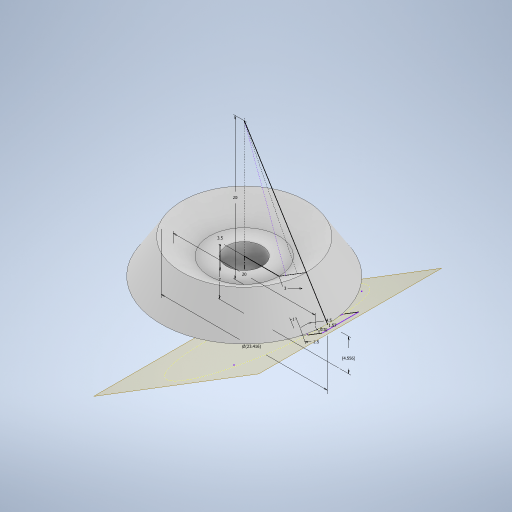
# Autodesk Inventor part: 베벨기어 002
Saved by Autodesk Inventor 2023 (Build 270158000, 158)
## iProperties
Created: 2022-06-18
Part Number: 베벨기어 002
Material: 일반
Document SubType Name: Modeling
Designer: fly01
Density: 1 g/cm^3
Appearance: 기본값
Author: fly01
Autodesk Inventor part; units mm, degrees
ref_plane "YZ Plane" through (0, 0, 0) normal (1, 0, 0) x (0, 1, 0)
ref_plane "XZ Plane" through (0, 0, 0) normal (0, 1, 0) x (-1, 0, 0)
ref_plane "XY Plane" through (0, 0, 0) normal (0, 0, 1) x (1, 0, 0)
sketch "스케치1" plane through (0, 0, 0) normal (0, 0, 1) x (1, 0, 0)
  line L0 (-10, 0) -> (10, 0) construction
  line L1 (0, 0) -> (0, 20) construction
  line L2 (0, 20) -> (10, 0) construction
  line L3 (0, 20) -> (11.7082, 1.0557)
  line L4 (0, 20) -> (5.8657, 4.0994) construction
  line L5 (7.8647, -1.3197) -> (11.7082, 1.0557)
  line L6 (7.8647, -1.3197) -> (7.0141, -1.8454)
  line L7 (7.0141, -1.8454) -> (3.9324, -1.8454)
  line L8 (3.9324, -1.8454) -> (3.9324, -3.5)
  line L9 (3.9324, -3.5) -> (0, -3.5)
  line L10 (8.7322, 5.871) -> (4.8959, 3.5)
  line L11 (4.8959, 3.5) -> (0, 3.5)
  line L12 (0, 3.5) -> (0, -3.5)
  line L13 (5.8657, 4.0994) -> (7.8647, -1.3197)
  point P0 (5.8657, 4.0994)
  dimension "d0" = 20
  dimension "d1" = 20
  dimension "d4" = 2
  dimension "d5" = 2.5
  dimension "d6" = 1
  dimension "d8" = 3
  dimension "d11" = 3.5
  dimension "d12" = 7
  dimension "d40" = 4.5557
  dimension "d41" = 23.4164
  constraints: 29 end point, 5 perpendicular, 5 point on line, 2 coincident, 2 horizontal, 1 collinear, 1 midpoint, 1 vertical
  measures "d0" distance of L0.start L0.end
  measures "d1" distance of L1.start L1.end
  measures "d4" distance from line of L3.end L2
  measures "d5" distance from line of L5.start L2
  measures "d6" distance of L5.start L6.end
  measures "d8" distance from line of L10.end L2
  measures "d11" distance between parallel lines of L0 L11
  measures "d12" distance between parallel lines of L11 L9
  measures "d40" distance from line of L9 L3.end
  measures "d41" diameter of L3.end L12
revolve "회전1" add sketch "스케치1" angle 360 about axis through (0, 3.5, 0) along (0, -1, 0)
sketch "스케치4" plane through (0, 3.5, 0) normal (0, 1, 0) x (1, 0, 0)
  circle A0 centre (0, 0) radius 2.5
  dimension "d35" = 5
  constraints: 1 centre point, 1 coincident
  measures "d35" diameter of A0
extrude "돌출1" cut sketch "스케치4" against normal blind 30.75
ref_plane "작업 평면4" through (7.8647, -1.3197, 0) normal (-0.5257, 0.8507, 0) x (-0.8507, -0.5257, 0)
sketch "스케치9" plane through (7.8647, -1.3197, 0) normal (-0.5257, 0.8507, 0) x (-0.8507, -0.5257, 0)
  ellipse E0 centre (5.4413, 0) end of major axis (5.4413, 11.7082) minor radius 9.9596 construction
  ellipse E1 centre (5.4413, 0) end of major axis (5.4413, 7.2082) minor radius 5.4596 (0.3405, 2.57) -> (0.0422, -1.07) ccw
  line L0 (-4.5183, 0) -> (-0.0183, 0)
  line L1 (-5.127, 1.07) -> (2.577, 1.07) construction
  line L2 (-5.5914, 1.57) -> (2.9534, 1.57) construction
  line L3 (-5.0964, 2.57) -> (1.9809, 2.57) construction
  arc A0 (-4.2754, 2.57) -> (0.0422, 1.07) centre (0.3783, 9.0013) ccw
  arc A1 (0.0422, -1.07) -> (-4.2754, -2.57) centre (0.3783, -9.0013) ccw
  line L4 (-4.2754, 2.57) -> (-6.6392, 2.57)
  line L5 (-6.6392, 2.57) -> (-6.6392, -2.57)
  line L6 (-6.6392, -2.57) -> (-4.2754, -2.57)
  point P0 (5.9964, 0)
  dimension "d55" = 1.57
  dimension "d56" = 4.5
  dimension "d57" = 0.5
  dimension "d58" = 1
  constraints: 14 end point, 4 point on circle, 4 point on line, 3 horizontal, 3 symmetric about line, 2 centre point, 2 perpendicular, 1 horizontal alignment, 10 other
  measures "d55" distance between parallel lines of L0 L2
  measures "d56" distance of L0.start L0.end
  measures "d57" distance between parallel lines of L2 L1
  measures "d58" distance between parallel lines of L3 L2
